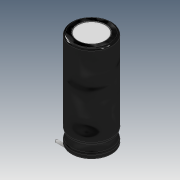
# Autodesk Inventor part: capacitor
Saved by Autodesk Inventor 2020 (Build 240168000, 168)
## iProperties
Created: 2020-09-27
Part Number: capacitor
Material: Generic
Document SubType Name: Modeling
Designer: DELL
Density: 1 g/cm^3
Appearance: Default
Author: DELL
Autodesk Inventor part; units mm, degrees
ref_plane "YZ Plane" through (0, 0, 0) normal (1, 0, 0) x (0, 1, 0)
ref_plane "XZ Plane" through (0, 0, 0) normal (0, 1, 0) x (-1, 0, 0)
sketch "Sketch1" plane through (0, 0, 0) normal (0, 0, 1) x (1, 0, 0)
  line L0 (0, 0) -> (-5.1, 0)
  line L1 (-5.1, 24.3) -> (-3.5, 24.3)
  line L2 (0, 24.2) -> (0, 0)
  line L3 (0, 0) -> (0, 14.6949)
  line L4 (-3.5, 24.3) -> (-3.5, 24.2)
  line L5 (-3.5, 24.2) -> (0, 24.2)
  spline S0 degree 2 poles (-5.1, 1.3) (-4.3, 2.4) (-5.1, 3.5) knots 0 0 0 1 1 1
  line L6 (-5.1, 0) -> (-5.1, 1.3)
  line L7 (-5.1, 3.5) -> (-5.1, 24.3)
  point P0 (-4.7, 2.4)
  dimension "d1" = 24.3
  dimension "d2" = 3.5
  dimension "d3" = 0.1
  dimension "d4" = 1.3
  dimension "d5" = 3.5
  dimension "d7" = 1.1
  constraints: 16 end point, 3 parallel, 2 perpendicular, 1 horizontal, 1 vertical, 5 other
  measures "d1" distance between parallel lines of L0 L1
  measures "d2" distance between parallel lines of L2 L4
  measures "d3" distance between parallel lines of L1 L5
  measures "d4" distance from line of L0 L6.end
  measures "d5" distance from line of L0 L7.start
  measures "d7" vertical distance of L6.end point (-4.7, 2.4)
revolve "Revolution1" add sketch "Sketch1" angle 360 about axis through (0, 0, 0) along (0, 1, 0)
fillet "Fillet1" radius 0.1 2 edges at (3.5, 24.3, 0) (3.5, 24.2, 0)
fillet "Fillet2" radius 0.5 1 edges at (5.1, 24.3, 0)
fillet "Fillet3" radius 1 2 edges at (5.1, 3.5, 0) (5.1, 1.3, 0)
fillet "Fillet4" radius 0.3 1 edges at (5.1, 0, 0)
sketch "Sketch2" plane through (0, 0, 0) normal (0, -1, 0) x (1, 0, 0)
  circle A0 centre (0, 2.9) radius 0.35
  circle A1 centre (0, -2.9) radius 0.35
  circle A2 centre (0, 0) radius 4.8 projected
  line L0 (-4.8, 0) -> (4.8, 0) construction
  line L1 (0, 4.8) -> (0, -4.8) construction
  dimension "d13" = 5.8
  dimension "d14" = 0.7
  constraints: 4 end point, 4 point on circle, 3 midpoint, 2 centre point, 1 horizontal, 1 point on line, 1 vertical, 1 other
  measures "d13" distance of A1.centre A0.centre
  measures "d14" diameter of A0
ref_plane "Work Plane1" through (0, 0, 2.9) normal (0, 0, 1) x (1, 0, 0)
sketch "Sketch3" plane through (0, 0, 2.9) normal (0, 0, 1) x (1, 0, 0)
  line L0 (-0.35, 0) -> (0.35, 0) projected
  line L1 (4.8, 0) -> (-4.8, 0) projected
  arc A0 (-1, -1) -> (0, 0) centre (-1, 0) ccw
  line L2 (-1, 0) -> (-1, -1) construction
  line L3 (-1, 0) -> (0, 0) construction
  line L4 (-1, -1) -> (-6, -1)
  point P0 (0, 0)
  dimension "d15" = 90
  dimension "d16" = 1
  dimension "d17" = 5
  constraints: 6 end point, 2 point on circle, 1 centre point, 1 horizontal, 1 point on line
  measures "d15" angle of L2 L3
  measures "d16" distance between parallel lines of L1 L4
  measures "d17" distance of L2.end L4.end
sweep "Sweep1" add profiles "Sketch2" path "Sketch3" path curves A0 L4 contours A0
mirror "Mirror1" about plane through (0, 0, 0) normal (0, 0, 1) of "Sweep1"
body "Solid1"
